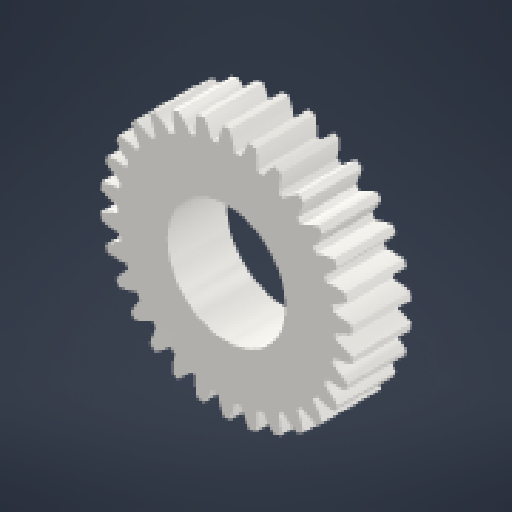
# Autodesk Inventor part: Spur Gear2
Saved by Autodesk Inventor 2025 (Build 290162000, 162)
## iProperties
CustomPartVersion: 1
Created: 2024-04-15
Part Number: Spur Gear2
Material: Steel
Document SubType Name: Modeling
Designer: sicia
Categories: <?xml version="1.0" encoding="UTF-16"?> <MemberInstance><Categories><FamilyTemplate><FamilyTemplateParameter ValueType="xs:double" Id="1" ObjectReferenceKey="da_z" ObjectType="kUserParameterObject"/><FamilyTemplateParameter ValueType="xs:double" Id="2" ObjectReferenceKey="da_b" ObjectType="kUserParameterObject"/><FamilyTemplateParameter ValueType="xs:double" Id="3" ObjectReferenceKey="da_beta" ObjectType="kUserParameterObject"/><FamilyTemplateParameter ValueType="xs:double" Id="4" ObjectReferenceKey="da_da" ObjectType="kUserParameterObject"/><FamilyTemplateParameter ValueType="xs:double" Id="5" ObjectReferenceKey="da_aw" ObjectType="kUserParameterObject"/><FamilyTemplateParameter ValueType="xs:string" Id="6" ObjectReferenceKey="EAIAABAAAACIAQAAAAAAAIAAAAAAAAAA" ObjectType="83910656" SubObjectId="SurfaceGeometry"/></FamilyTemplate><ParamToTemplateMap><ParamToTemplate CategoryParameter="//CategoryParameter[@InternalName='046C89C9-8512-4d59-83FE-43B91F4F132A']" TemplateParameter="1"/><ParamToTemplate CategoryParameter="//CategoryParameter[@InternalName='2552DF32-E462-4b46-AEBF-C6C7768E72AC']" TemplateParameter="2"/><ParamToTemplate CategoryParameter="//CategoryParameter[@InternalName='C9EE641D-15FC-4fae-A226-E94C4372FDD7']" TemplateParameter="3"/><ParamToTemplate><ParamToTemplate CategoryParameter="//CategoryParameter[@InternalName='00B6519A-459B-49c7-AD84-2E56D39A5744']" ConstantValue="-0.395666"/></ParamToTemplate><ParamToTemplate><ParamToTemplate CategoryParameter="//CategoryParameter[@InternalName='04B31F0E-C7A6-4894-AA32-9629BEFACF47']" ConstantValue="1.000000"/></ParamToTemplate><ParamToTemplate><ParamToTemplate CategoryParameter="//CategoryParameter[@InternalName='43CBEC2E-7847-49e7-A936-2F7889FCB2D9']" ConstantValue="0.250000"/></ParamToTemplate><ParamToTemplate><ParamToTemplate CategoryParameter="//CategoryParameter[@InternalName='B1EFC894-105D-4ebd-86BF-FA20ED196853']" ConstantValue="0.333500"/></ParamToTemplate><ParamToTemplate><ParamToTemplate CategoryParameter="//CategoryParameter[@InternalName='51175063-3D10-4879-93E8-6246FE8B403D']" ConstantValue="2060000000.000000"/></ParamToTemplate><ParamToTemplate><ParamToTemplate CategoryParameter="//CategoryParameter[@InternalName='A3A52E27-4454-46a9-B0BD-C932399B70AF']" ConstantValue="0.300000"/></ParamToTemplate><ParamToTemplate><ParamToTemplate CategoryParameter="//CategoryParameter[@InternalName='91B76062-C214-41d9-B1B9-14D2AB99603D']" ConstantValue="0.137500"/></ParamToTemplate><ParamToTemplate><ParamToTemplate CategoryParameter="//CategoryParameter[@InternalName='374E806E-8B8A-4dda-A9AA-1039D6500AD2']" ConstantValue="7.272727"/></ParamToTemplate><ParamToTemplate><ParamToTemplate CategoryParameter="//CategoryParameter[@InternalName='2D373A89-B862-43d6-8D0B-0CBF12AB9F6C']" ConstantValue="0.349066"/></ParamToTemplate><ParamToTemplate CategoryParameter="//CategoryParameter[@InternalName='37777632-D6A2-4fac-9D53-DB8ACD95C989']" TemplateParameter="4"/><ParamToTemplate CategoryParameter="//CategoryParameter[@InternalName='FD1017F1-B727-4f7e-9707-0F86F1FF9423']" TemplateParameter="5"/><ParamToTemplate><ParamToTemplate CategoryParameter="//CategoryParameter[@InternalName='9E1B4470-B2D3-4ff1-B813-535BB4CDF51A']" ConstantValue="3520000.000000"/></ParamToTemplate><ParamToTemplate><ParamToTemplate CategoryParameter="//CategoryParameter[@InternalName='F8452263-BFF6-458c-9FB1-07C4B99E95CD']" ConstantValue="11400000.000000"/></ParamToTemplate><ParamToTemplate><ParamToTemplate CategoryParameter="//CategoryParameter[@InternalName='3E3BB259-FD49-497f-8171-6EBC954A3479']" ConstantValue="2.000000"/></ParamToTemplate><ParamToTemplate CategoryParameter="//CategoryParameter[@InternalName='27C3BAF2-7550-4e4b-AE2C-0DB134B7D9B7']" TemplateParameter="6"/></ParamToTemplateMap><Category DisplayName="Gear" InternalName="DC85795E-93AB-48d5-8EEE-5A27447B64BD" Mnemonic="Gear"><CategoryParameter DisplayName="z" InternalName="046C89C9-8512-4d59-83FE-43B91F4F132A" Mnemonic="z"/><CategoryParameter DisplayName="b" InternalName="2552DF32-E462-4b46-AEBF-C6C7768E72AC" Mnemonic="b"/><CategoryParameter DisplayName="||b|" InternalName="C9EE641D-15FC-4fae-A226-E94C4372FDD7" Mnemonic="beta"/><CategoryParameter DisplayName="x" InternalName="00B6519A-459B-49c7-AD84-2E56D39A5744" Mnemonic="x"/><CategoryParameter DisplayName="a*" InternalName="04B31F0E-C7A6-4894-AA32-9629BEFACF47" Mnemonic="a"/><CategoryParameter DisplayName="c*" InternalName="43CBEC2E-7847-49e7-A936-2F7889FCB2D9" Mnemonic="c"/><CategoryParameter DisplayName="r|.f|*" InternalName="B1EFC894-105D-4ebd-86BF-FA20ED196853" Mnemonic="rf"/><CategoryParameter DisplayName="E" InternalName="51175063-3D10-4879-93E8-6246FE8B403D" Mnemonic="E"/><CategoryParameter DisplayName="||m|" InternalName="A3A52E27-4454-46a9-B0BD-C932399B70AF" Mnemonic="mi"/><Category DisplayName="SpurGear" InternalName="26C5A22E-A91E-4dfd-A3B3-23CCAFAE1764" Mnemonic="SpurGear"><CategoryParameter DisplayName="m" InternalName="91B76062-C214-41d9-B1B9-14D2AB99603D" Mnemonic="m"/><CategoryParameter DisplayName="P" InternalName="374E806E-8B8A-4dda-A9AA-1039D6500AD2" Mnemonic="PP"/><CategoryParameter DisplayName="||a|" InternalName="2D373A89-B862-43d6-8D0B-0CBF12AB9F6C" Mnemonic="alpha"/><CategoryParameter DisplayName="d|.a|" InternalName="37777632-D6A2-4fac-9D53-DB8ACD95C989" Mnemonic="da"/><CategoryParameter DisplayName="a|.w|" InternalName="FD1017F1-B727-4f7e-9707-0F86F1FF9423" Mnemonic="aw"/><CategoryParameter DisplayName="||s||.Flim|" InternalName="9E1B4470-B2D3-4ff1-B813-535BB4CDF51A" Mnemonic="sFlim"/><CategoryParameter DisplayName="||s||.Hlim|" InternalName="F8452263-BFF6-458c-9FB1-07C4B99E95CD" Mnemonic="sHlim"/><CategoryParameter DisplayName="type" InternalName="3E3BB259-FD49-497f-8171-6EBC954A3479" Mnemonic="type"/><CategoryParameter DisplayName="PitchDiameter" InternalName="27C3BAF2-7550-4e4b-AE2C-0DB134B7D9B7" Mnemonic="IDS_PITCHDIAM"/></Category></Category></Categories></MemberInstance>
Density: 7.85 g/cm^3
Appearance: Steel
Mass: 73.1894 g
Surface Area: 49.8599 cm^2
Volume: 9.32349 cm^3
Author: sicia
Autodesk Inventor part; units mm, degrees
sketch "Sketch1" plane through (0, 0, 0) normal (0, 0, 1) x (1, 0, 0)
  circle A0 centre (0, 0) radius 21.2941
  dimension "d0" = 42.5881
  constraints: 1 centre point
  measures "d0" diameter of A0
extrude "Extrusion1" add sketch "Sketch1" along normal blind 10
ref_plane "Work Plane2" through (0, 0, 5) normal (0, 0, 1) x (1, 0, 0)
sketch "Sketch2" plane through (0, 0, 0) normal (0, 0, -1) x (-1, 0, 0)
  circle A0 centre (0, 0) radius 21.2941 projected
  circle A1 centre (0, 0) radius 20.625
  dimension "d3" = 41.25
  constraints: 1 centre point, 1 coincident
  measures "d3" diameter of A1
surface extrude "Pitch Diameter" sketch "Sketch2" against normal through all shown no curves A1
ref_plane "Work Plane8" through (0, 0, 0) normal (0.9945219, 0.1045285, 0) x (0, 0, 1)
ref_plane "Work Plane9" through (0, 0, 0) normal (1, 0, 0) x (0, 1, 0)
spur gear teeth "Spur Gear" teeth 30 pitch diameter 41.25 tip diameter 42.5881 root diameter 36.7244 face width 10 start plane through (0, 0, 0) normal (0, 0, -1) x (-1, 0, 0)
sketch "Sketch3" plane through (0, 0, 0) normal (0, 0, -1) x (-1, 0, 0)
  circle A0 centre (0, 0) radius 10
  dimension "d49" = 20
  constraints: 1 centre point, 1 coincident
  measures "d49" diameter of A0
extrude "Extrusion2" cut sketch "Sketch3" against normal blind 10
sketch "Sketch4" plane through (0, 0, 0) normal (0, 0, -1) x (-1, 0, 0)
  circle A0 centre (0, 0) radius 10 projected
  arc A1 (5.2151, 17.606) -> (4.971, 20.7057) centre (-7.7232, 18.1464) ccw projected
  arc A2 (4.971, 20.7057) -> (3.8805, 20.9375) centre (0, 0) ccw projected
  arc A3 (3.8805, 20.9375) -> (2.3967, 18.2051) centre (14.4363, 13.4362) ccw projected
  arc A4 (2.3967, 18.2051) -> (1.4407, 18.3056) centre (0, 0) ccw projected
  arc A5 (1.4407, 18.3056) -> (0.5574, 21.2868) centre (-11.3273, 16.1441) ccw projected
  arc A6 (0.5574, 21.2868) -> (-0.5574, 21.2868) centre (0, 0) ccw projected
  arc A7 (-0.5574, 21.2868) -> (-1.4407, 18.3056) centre (11.3273, 16.1441) ccw projected
  arc A8 (-1.4407, 18.3056) -> (-2.3967, 18.2051) centre (0, 0) ccw projected
  arc A9 (-2.3967, 18.2051) -> (-3.8805, 20.9375) centre (-14.4363, 13.4362) ccw projected
  arc A10 (-3.8805, 20.9375) -> (-4.971, 20.7057) centre (0, 0) ccw projected
  arc A11 (-4.971, 20.7057) -> (-5.2151, 17.606) centre (7.7232, 18.1464) ccw projected
  arc A12 (-5.2151, 17.606) -> (-6.1294, 17.309) centre (0, 0) ccw projected
  arc A13 (-6.1294, 17.309) -> (-8.1489, 19.6731) centre (-16.9144, 10.1411) ccw projected
  arc A14 (-8.1489, 19.6731) -> (-9.1673, 19.2197) centre (0, 0) ccw projected
  arc A15 (-9.1673, 19.2197) -> (-8.7617, 16.137) centre (3.7816, 19.3556) ccw projected
  arc A16 (-8.7617, 16.137) -> (-9.5942, 15.6564) centre (0, 0) ccw projected
  arc A17 (-9.5942, 15.6564) -> (-12.0611, 17.549) centre (-18.6532, 6.4028) ccw projected
  arc A18 (-12.0611, 17.549) -> (-12.963, 16.8937) centre (0, 0) ccw projected
  arc A19 (-12.963, 16.8937) -> (-11.9253, 13.9627) centre (-0.3253, 19.7188) ccw projected
  arc A20 (-11.9253, 13.9627) -> (-12.6397, 13.3195) centre (0, 0) ccw projected
  arc A21 (-12.6397, 13.3195) -> (-15.4462, 14.6579) centre (-19.5768, 2.3847) ccw projected
  arc A22 (-15.4462, 14.6579) -> (-16.1921, 13.8294) centre (0, 0) ccw projected
  arc A23 (-16.1921, 13.8294) -> (-14.5677, 11.1782) centre (-4.418, 19.2203) ccw projected
  arc A24 (-14.5677, 11.1782) -> (-15.1328, 10.4005) centre (0, 0) ccw projected
  arc A25 (-15.1328, 10.4005) -> (-18.1562, 11.1261) centre (-19.6448, -1.7377) ccw projected
  arc A26 (-18.1562, 11.1261) -> (-18.7136, 10.1606) centre (0, 0) ccw projected
  arc A27 (-18.7136, 10.1606) -> (-16.5735, 7.9051) centre (-8.3176, 17.8817) ccw projected
  arc A28 (-16.5735, 7.9051) -> (-16.9645, 7.0269) centre (0, 0) ccw projected
  arc A29 (-16.9645, 7.0269) -> (-20.0727, 7.1081) centre (-18.8543, -5.7841) ccw projected
  arc A30 (-20.0727, 7.1081) -> (-20.4172, 6.0478) centre (0, 0) ccw projected
  arc A31 (-20.4172, 6.0478) -> (-17.8549, 4.2866) centre (-11.8536, 15.7617) ccw projected
  arc A32 (-17.8549, 4.2866) -> (-18.0547, 3.3462) centre (0, 0) ccw projected
  arc A33 (-18.0547, 3.3462) -> (-21.1119, 2.7794) centre (-17.2397, -9.5777) ccw projected
  arc A34 (-21.1119, 2.7794) -> (-21.2284, 1.6707) centre (0, 0) ccw projected
  arc A35 (-21.2284, 1.6707) -> (-18.3559, 0.4807) centre (-14.8716, 12.9527) ccw projected
  arc A36 (-18.3559, 0.4807) -> (-18.3559, -0.4807) centre (0, 0) ccw projected
  arc A37 (-18.3559, -0.4807) -> (-21.2284, -1.6707) centre (-14.8716, -12.9527) ccw projected
  arc A38 (-21.2284, -1.6707) -> (-21.1119, -2.7794) centre (0, 0) ccw projected
  arc A39 (-21.1119, -2.7794) -> (-18.0547, -3.3462) centre (-17.2397, 9.5777) ccw projected
  arc A40 (-18.0547, -3.3462) -> (-17.8549, -4.2866) centre (0, 0) ccw projected
  arc A41 (-17.8549, -4.2866) -> (-20.4172, -6.0478) centre (-11.8536, -15.7617) ccw projected
  arc A42 (-20.4172, -6.0478) -> (-20.0727, -7.1081) centre (0, 0) ccw projected
  arc A43 (-20.0727, -7.1081) -> (-16.9645, -7.0269) centre (-18.8543, 5.7841) ccw projected
  arc A44 (-16.9645, -7.0269) -> (-16.5735, -7.9051) centre (0, 0) ccw projected
  arc A45 (-16.5735, -7.9051) -> (-18.7136, -10.1606) centre (-8.3176, -17.8817) ccw projected
  arc A46 (-18.7136, -10.1606) -> (-18.1562, -11.1261) centre (0, 0) ccw projected
  arc A47 (-18.1562, -11.1261) -> (-15.1328, -10.4005) centre (-19.6448, 1.7377) ccw projected
  arc A48 (-15.1328, -10.4005) -> (-14.5677, -11.1782) centre (0, 0) ccw projected
  arc A49 (-14.5677, -11.1782) -> (-16.1921, -13.8294) centre (-4.418, -19.2203) ccw projected
  arc A50 (-16.1921, -13.8294) -> (-15.4462, -14.6579) centre (0, 0) ccw projected
  arc A51 (-15.4462, -14.6579) -> (-12.6397, -13.3195) centre (-19.5768, -2.3847) ccw projected
  arc A52 (-12.6397, -13.3195) -> (-11.9253, -13.9627) centre (0, 0) ccw projected
  arc A53 (-11.9253, -13.9627) -> (-12.963, -16.8937) centre (-0.3253, -19.7188) ccw projected
  arc A54 (-12.963, -16.8937) -> (-12.0611, -17.549) centre (0, 0) ccw projected
  arc A55 (-12.0611, -17.549) -> (-9.5942, -15.6564) centre (-18.6532, -6.4028) ccw projected
  arc A56 (-9.5942, -15.6564) -> (-8.7617, -16.137) centre (0, 0) ccw projected
  arc A57 (-8.7617, -16.137) -> (-9.1673, -19.2197) centre (3.7816, -19.3556) ccw projected
  arc A58 (-9.1673, -19.2197) -> (-8.1489, -19.6731) centre (0, 0) ccw projected
  arc A59 (-8.1489, -19.6731) -> (-6.1294, -17.309) centre (-16.9144, -10.1411) ccw projected
  arc A60 (-6.1294, -17.309) -> (-5.2151, -17.606) centre (0, 0) ccw projected
  arc A61 (-5.2151, -17.606) -> (-4.971, -20.7057) centre (7.7232, -18.1464) ccw projected
  arc A62 (-4.971, -20.7057) -> (-3.8805, -20.9375) centre (0, 0) ccw projected
  arc A63 (-3.8805, -20.9375) -> (-2.3967, -18.2051) centre (-14.4363, -13.4362) ccw projected
  arc A64 (-2.3967, -18.2051) -> (-1.4407, -18.3056) centre (0, 0) ccw projected
  arc A65 (-1.4407, -18.3056) -> (-0.5574, -21.2868) centre (11.3273, -16.1441) ccw projected
  arc A66 (-0.5574, -21.2868) -> (0.5574, -21.2868) centre (0, 0) ccw projected
  arc A67 (0.5574, -21.2868) -> (1.4407, -18.3056) centre (-11.3273, -16.1441) ccw projected
  arc A68 (1.4407, -18.3056) -> (2.3967, -18.2051) centre (0, 0) ccw projected
  arc A69 (2.3967, -18.2051) -> (3.8805, -20.9375) centre (14.4363, -13.4362) ccw projected
  arc A70 (3.8805, -20.9375) -> (4.971, -20.7057) centre (0, 0) ccw projected
  arc A71 (4.971, -20.7057) -> (5.2151, -17.606) centre (-7.7232, -18.1464) ccw projected
  arc A72 (5.2151, -17.606) -> (6.1294, -17.309) centre (0, 0) ccw projected
  arc A73 (6.1294, -17.309) -> (8.1489, -19.6731) centre (16.9144, -10.1411) ccw projected
  arc A74 (8.1489, -19.6731) -> (9.1673, -19.2197) centre (0, 0) ccw projected
  arc A75 (9.1673, -19.2197) -> (8.7617, -16.137) centre (-3.7816, -19.3556) ccw projected
  arc A76 (8.7617, -16.137) -> (9.5942, -15.6564) centre (0, 0) ccw projected
  arc A77 (9.5942, -15.6564) -> (12.0611, -17.549) centre (18.6532, -6.4028) ccw projected
  arc A78 (12.0611, -17.549) -> (12.963, -16.8937) centre (0, 0) ccw projected
  arc A79 (12.963, -16.8937) -> (11.9253, -13.9627) centre (0.3253, -19.7188) ccw projected
  arc A80 (11.9253, -13.9627) -> (12.6397, -13.3195) centre (0, 0) ccw projected
  arc A81 (12.6397, -13.3195) -> (15.4462, -14.6579) centre (19.5768, -2.3847) ccw projected
  arc A82 (15.4462, -14.6579) -> (16.1921, -13.8294) centre (0, 0) ccw projected
  arc A83 (16.1921, -13.8294) -> (14.5677, -11.1782) centre (4.418, -19.2203) ccw projected
  arc A84 (14.5677, -11.1782) -> (15.1328, -10.4005) centre (0, 0) ccw projected
  arc A85 (15.1328, -10.4005) -> (18.1562, -11.1261) centre (19.6448, 1.7377) ccw projected
  arc A86 (18.1562, -11.1261) -> (18.7136, -10.1606) centre (0, 0) ccw projected
  arc A87 (18.7136, -10.1606) -> (16.5735, -7.9051) centre (8.3176, -17.8817) ccw projected
  arc A88 (16.5735, -7.9051) -> (16.9645, -7.0269) centre (0, 0) ccw projected
  arc A89 (16.9645, -7.0269) -> (20.0727, -7.1081) centre (18.8543, 5.7841) ccw projected
  arc A90 (20.0727, -7.1081) -> (20.4172, -6.0478) centre (0, 0) ccw projected
  arc A91 (20.4172, -6.0478) -> (17.8549, -4.2866) centre (11.8536, -15.7617) ccw projected
  arc A92 (17.8549, -4.2866) -> (18.0547, -3.3462) centre (0, 0) ccw projected
  arc A93 (18.0547, -3.3462) -> (21.1119, -2.7794) centre (17.2397, 9.5777) ccw projected
  arc A94 (21.1119, -2.7794) -> (21.2284, -1.6707) centre (0, 0) ccw projected
  arc A95 (21.2284, -1.6707) -> (18.3559, -0.4807) centre (14.8716, -12.9527) ccw projected
  arc A96 (18.3559, -0.4807) -> (18.3559, 0.4807) centre (0, 0) ccw projected
  arc A97 (18.3559, 0.4807) -> (21.2284, 1.6707) centre (14.8716, 12.9527) ccw projected
  arc A98 (21.2284, 1.6707) -> (21.1119, 2.7794) centre (0, 0) ccw projected
  arc A99 (21.1119, 2.7794) -> (18.0547, 3.3462) centre (17.2397, -9.5777) ccw projected
  arc A100 (18.0547, 3.3462) -> (17.8549, 4.2866) centre (0, 0) ccw projected
  arc A101 (17.8549, 4.2866) -> (20.4172, 6.0478) centre (11.8536, 15.7617) ccw projected
  arc A102 (20.4172, 6.0478) -> (20.0727, 7.1081) centre (0, 0) ccw projected
  arc A103 (20.0727, 7.1081) -> (16.9645, 7.0269) centre (18.8543, -5.7841) ccw projected
  arc A104 (16.9645, 7.0269) -> (16.5735, 7.9051) centre (0, 0) ccw projected
  arc A105 (16.5735, 7.9051) -> (18.7136, 10.1606) centre (8.3176, 17.8817) ccw projected
  arc A106 (18.7136, 10.1606) -> (18.1562, 11.1261) centre (0, 0) ccw projected
  arc A107 (18.1562, 11.1261) -> (15.1328, 10.4005) centre (19.6448, -1.7377) ccw projected
  arc A108 (15.1328, 10.4005) -> (14.5677, 11.1782) centre (0, 0) ccw projected
  arc A109 (14.5677, 11.1782) -> (16.1921, 13.8294) centre (4.418, 19.2203) ccw projected
  arc A110 (16.1921, 13.8294) -> (15.4462, 14.6579) centre (0, 0) ccw projected
  arc A111 (15.4462, 14.6579) -> (12.6397, 13.3195) centre (19.5768, 2.3847) ccw projected
  arc A112 (12.6397, 13.3195) -> (11.9253, 13.9627) centre (0, 0) ccw projected
  arc A113 (11.9253, 13.9627) -> (12.963, 16.8937) centre (0.3253, 19.7188) ccw projected
  arc A114 (12.963, 16.8937) -> (12.0611, 17.549) centre (0, 0) ccw projected
  arc A115 (12.0611, 17.549) -> (9.5942, 15.6564) centre (18.6532, 6.4028) ccw projected
  arc A116 (9.5942, 15.6564) -> (8.7617, 16.137) centre (0, 0) ccw projected
  arc A117 (8.7617, 16.137) -> (9.1673, 19.2197) centre (-3.7816, 19.3556) ccw projected
  arc A118 (9.1673, 19.2197) -> (8.1489, 19.6731) centre (0, 0) ccw projected
  arc A119 (8.1489, 19.6731) -> (6.1294, 17.309) centre (16.9144, 10.1411) ccw projected
  arc A120 (6.1294, 17.309) -> (5.2151, 17.606) centre (0, 0) ccw projected
equation "\"d0\" = da_da"
equation "\"d1\" = da_b"
equation "\"d3\" = da_d"
equation "\"d16\" = da_aw"
equation "\"d43\" = da_aw"
equation "\"d46\" = da_aw"
equation "\"da_da\" = 42.588104"
equation "\"da_b\" = 10"
equation "\"da_d\" = 41.25"
equation "\"da_aw\" = 40.000011"
body "Solid1"
body "Srf1"
